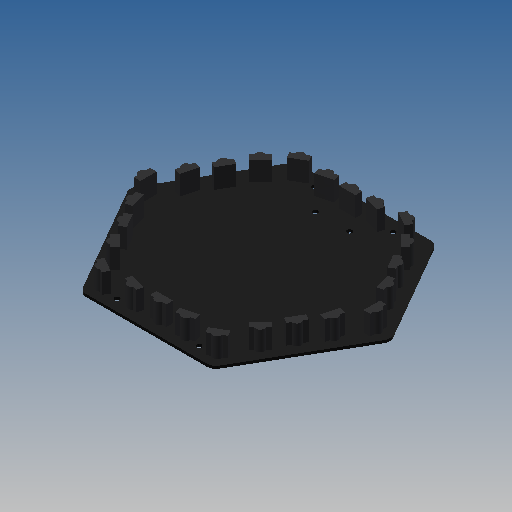
# Autodesk Inventor part: PCB
Saved by Autodesk Inventor 2017 (Build 210142000, 142)
## iProperties
Created: 2016-10-01
Part Number: PCB
Material: Generic
Document SubType Name: Modeling
Designer: James Yelland
Density: 1 g/cm^3
Appearance: Default
Mass: 32.3214 g
Surface Area: 333.79 cm^2
Volume: 32.3214 cm^3
Author: James Yelland
Autodesk Inventor part; units mm, degrees
ref_plane "YZ Plane" through (0, 0, 0) normal (1, 0, 0) x (0, 1, 0)
ref_plane "XZ Plane" through (0, 0, 0) normal (0, 1, 0) x (-1, 0, 0)
ref_plane "XY Plane" through (0, 0, 0) normal (0, 0, 1) x (1, 0, 0)
sketch "Sketch1" plane through (0, 0, 0) normal (0, 1, 0) x (-1, 0, 0)
  line L0 (-78.5566, 2.5) -> (-41.4434, 66.782)
  line L1 (-37.1132, 69.282) -> (37.1132, 69.282)
  line L2 (41.4434, 66.782) -> (78.5566, 2.5)
  line L3 (0, -64.282) -> (-40, -64.282)
  line L4 (0, -64.282) -> (40, -64.282)
  line L5 (78.5566, -2.5) -> (44.3301, -61.782)
  line L6 (-44.3301, -61.782) -> (-78.5566, -2.5)
  arc A0 (78.5566, -2.5) -> (78.5566, 2.5) centre (74.2265, 0) ccw
  arc A1 (40, -64.282) -> (44.3301, -61.782) centre (40, -59.282) ccw
  arc A2 (-44.3301, -61.782) -> (-40, -64.282) centre (-40, -59.282) ccw
  arc A3 (-78.5566, 2.5) -> (-78.5566, -2.5) centre (-74.2265, 0) ccw
  arc A4 (-37.1132, 69.282) -> (-41.4434, 66.782) centre (-37.1132, 64.282) ccw
  arc A5 (41.4434, 66.782) -> (37.1132, 69.282) centre (37.1132, 64.282) ccw
  point P0 (80, 0)
  point P1 (-80, 0)
  point P2 (-42.8868, -64.282)
  point P3 (42.8868, -64.282)
  dimension "d21" = 5
  constraints: 14 end point, 12 point on circle, 12 tangent, 9 point on line, 6 centre point, 5 equal radius
  measures "d21" radius of A0
extrude "Extrusion1" add sketch "Sketch1" along normal blind 1.6
sketch "Sketch4" plane through (0, 1.6, 0) normal (0, 1, 0) x (1, 0, 0)
  line L0 (5, 57.282) -> (5, 53.282)
  arc A0 (2.5807, 57.282) -> (-2.5807, 57.282) centre (0, 56.332) ccw
  line L1 (-5, 57.282) -> (-2.5807, 57.282)
  line L2 (5, 53.282) -> (-5, 53.282)
  line L3 (-5, 53.282) -> (-5, 57.282)
  line L4 (2.5807, 57.282) -> (5, 57.282)
  line L5 (40, 64.282) -> (-40, 64.282)
  arc A1 (-40, 64.282) -> (-44.3301, 61.782) centre (-40, 59.282) ccw
  line L6 (-44.3301, 61.782) -> (-78.5566, 2.5)
  arc A2 (-78.5566, 2.5) -> (-78.5566, -2.5) centre (-74.2265, 0) ccw
  line L7 (-78.5566, -2.5) -> (-41.4434, -66.782)
  arc A3 (-41.4434, -66.782) -> (-37.1132, -69.282) centre (-37.1132, -64.282) ccw
  line L8 (-37.1132, -69.282) -> (37.1132, -69.282)
  arc A4 (37.1132, -69.282) -> (41.4434, -66.782) centre (37.1132, -64.282) ccw
  line L9 (41.4434, -66.782) -> (78.5566, -2.5)
  arc A5 (78.5566, -2.5) -> (78.5566, 2.5) centre (74.2265, 0) ccw
  line L10 (78.5566, 2.5) -> (44.3301, 61.782)
  arc A6 (44.3301, 61.782) -> (40, 64.282) centre (40, 59.282) ccw
  line L11 (0, 56.332) -> (0, 64.282)
  line L12 (-19.2069, 52.3628) -> (-20.2422, 56.2265)
  line L13 (-20.2422, 56.2265) -> (-17.9053, 56.8526)
  arc A7 (-12.9198, 58.1885) -> (-17.9053, 56.8526) centre (-15.1667, 56.6029) ccw
  line L14 (-9.5477, 54.9509) -> (-19.2069, 52.3628)
  line L15 (-10.583, 58.8146) -> (-9.5477, 54.9509)
  line L16 (-12.9198, 58.1885) -> (-10.583, 58.8146)
  line L17 (-15.1667, 56.6029) -> (-17.2243, 64.282)
  line L18 (-35.9434, 52.2558) -> (-37.9434, 55.7199)
  line L19 (-37.9434, 55.7199) -> (-35.8482, 56.9295)
  arc A8 (-31.3783, 59.5102) -> (-35.8482, 56.9295) centre (-33.1382, 57.3971) ccw
  line L20 (-27.2831, 57.2558) -> (-35.9434, 52.2558)
  line L21 (-29.2831, 60.7199) -> (-27.2831, 57.2558)
  line L22 (-31.3783, 59.5102) -> (-29.2831, 60.7199)
  line L23 (-33.1382, 57.3971) -> (-37.1132, 64.282)
  line L24 (-46.4753, 39.4043) -> (-49.3038, 42.2327)
  line L25 (-49.3038, 42.2327) -> (-47.593, 43.9434)
  arc A9 (-43.9434, 47.593) -> (-47.593, 43.9434) centre (-45.0965, 45.0965) ccw
  line L26 (-39.4043, 46.4753) -> (-46.4753, 39.4043)
  line L27 (-42.2327, 49.3038) -> (-39.4043, 46.4753)
  line L28 (-43.9434, 47.593) -> (-42.2327, 49.3038)
  line L29 (-45.0965, 45.0965) -> (-50.718, 50.718)
  line L30 (-52.9737, 24.8109) -> (-56.4378, 26.8109)
  line L31 (-56.4378, 26.8109) -> (-55.2282, 28.9061)
  arc A10 (-52.6475, 33.376) -> (-55.2282, 28.9061) centre (-53.1151, 30.666) ccw
  line L32 (-47.9737, 33.4711) -> (-52.9737, 24.8109)
  line L33 (-51.4378, 35.4711) -> (-47.9737, 33.4711)
  line L34 (-52.6475, 33.376) -> (-51.4378, 35.4711)
  line L35 (-53.1151, 30.666) -> (-60, 34.641)
  line L36 (-59.9509, 10.8874) -> (-63.8146, 11.9227)
  line L37 (-63.8146, 11.9227) -> (-63.1885, 14.2596)
  arc A11 (-61.8526, 19.2451) -> (-63.1885, 14.2596) centre (-61.6029, 16.5065) ccw
  line L38 (-57.3628, 20.5467) -> (-59.9509, 10.8874)
  line L39 (-61.2265, 21.582) -> (-57.3628, 20.5467)
  line L40 (-61.8526, 19.2451) -> (-61.2265, 21.582)
  line L41 (-61.6029, 16.5065) -> (-69.282, 18.5641)
  line L42 (-68.2265, -5) -> (-72.2265, -5)
  line L43 (-72.2265, -5) -> (-72.2265, -2.5807)
  arc A12 (-72.2265, 2.5807) -> (-72.2265, -2.5807) centre (-71.2765, 0) ccw
  line L44 (-68.2265, 5) -> (-68.2265, -5)
  line L45 (-72.2265, 5) -> (-68.2265, 5)
  line L46 (-72.2265, 2.5807) -> (-72.2265, 5)
  line L47 (-71.2765, 0) -> (-79.2265, 0)
  line L48 (-57.3628, -20.5467) -> (-61.2265, -21.582)
  line L49 (-61.2265, -21.582) -> (-61.8526, -19.2451)
  arc A13 (-63.1885, -14.2596) -> (-61.8526, -19.2451) centre (-61.6029, -16.5065) ccw
  line L50 (-59.9509, -10.8874) -> (-57.3628, -20.5467)
  line L51 (-63.8146, -11.9227) -> (-59.9509, -10.8874)
  line L52 (-63.1885, -14.2596) -> (-63.8146, -11.9227)
  line L53 (-61.6029, -16.5065) -> (-69.282, -18.5641)
  line L54 (-47.9737, -33.4711) -> (-51.4378, -35.4711)
  line L55 (-51.4378, -35.4711) -> (-52.6475, -33.376)
  arc A14 (-55.2282, -28.9061) -> (-52.6475, -33.376) centre (-53.1151, -30.666) ccw
  line L56 (-52.9737, -24.8109) -> (-47.9737, -33.4711)
  line L57 (-56.4378, -26.8109) -> (-52.9737, -24.8109)
  line L58 (-55.2282, -28.9061) -> (-56.4378, -26.8109)
  line L59 (-53.1151, -30.666) -> (-60, -34.641)
  line L60 (-39.4043, -46.4753) -> (-42.2327, -49.3038)
  line L61 (-42.2327, -49.3038) -> (-43.9434, -47.593)
  arc A15 (-47.593, -43.9434) -> (-43.9434, -47.593) centre (-45.0965, -45.0965) ccw
  line L62 (-46.4753, -39.4043) -> (-39.4043, -46.4753)
  line L63 (-49.3038, -42.2327) -> (-46.4753, -39.4043)
  line L64 (-47.593, -43.9434) -> (-49.3038, -42.2327)
  line L65 (-45.0965, -45.0965) -> (-50.718, -50.718)
  line L66 (-29.7831, -61.5859) -> (-31.7831, -65.05)
  line L67 (-31.7831, -65.05) -> (-33.8783, -63.8403)
  arc A16 (-38.3482, -61.2596) -> (-33.8783, -63.8403) centre (-35.6382, -61.7273) ccw
  line L68 (-38.4434, -56.5859) -> (-29.7831, -61.5859)
  line L69 (-40.4434, -60.05) -> (-38.4434, -56.5859)
  line L70 (-38.3482, -61.2596) -> (-40.4434, -60.05)
  line L71 (-35.6382, -61.7273) -> (-39.6132, -68.6122)
  line L72 (-10.8874, -59.9509) -> (-11.9227, -63.8146)
  line L73 (-11.9227, -63.8146) -> (-14.2596, -63.1885)
  arc A17 (-19.2451, -61.8526) -> (-14.2596, -63.1885) centre (-16.5065, -61.6029) ccw
  line L74 (-20.5467, -57.3628) -> (-10.8874, -59.9509)
  line L75 (-21.582, -61.2265) -> (-20.5467, -57.3628)
  line L76 (-19.2451, -61.8526) -> (-21.582, -61.2265)
  line L77 (-16.5065, -61.6029) -> (-18.5641, -69.282)
  line L78 (5, -58.282) -> (5, -62.282)
  line L79 (5, -62.282) -> (2.5807, -62.282)
  arc A18 (-2.5807, -62.282) -> (2.5807, -62.282) centre (0, -61.332) ccw
  line L80 (-5, -58.282) -> (5, -58.282)
  line L81 (-5, -62.282) -> (-5, -58.282)
  line L82 (-2.5807, -62.282) -> (-5, -62.282)
  line L83 (0, -61.332) -> (0, -69.282)
  line L84 (20.5467, -57.3628) -> (21.582, -61.2265)
  line L85 (21.582, -61.2265) -> (19.2451, -61.8526)
  arc A19 (14.2596, -63.1885) -> (19.2451, -61.8526) centre (16.5065, -61.6029) ccw
  line L86 (10.8874, -59.9509) -> (20.5467, -57.3628)
  line L87 (11.9227, -63.8146) -> (10.8874, -59.9509)
  line L88 (14.2596, -63.1885) -> (11.9227, -63.8146)
  line L89 (16.5065, -61.6029) -> (18.5641, -69.282)
  line L90 (38.4434, -56.5859) -> (40.4434, -60.05)
  line L91 (40.4434, -60.05) -> (38.3482, -61.2596)
  arc A20 (33.8783, -63.8403) -> (38.3482, -61.2596) centre (35.6382, -61.7273) ccw
  line L92 (29.7831, -61.5859) -> (38.4434, -56.5859)
  line L93 (31.7831, -65.05) -> (29.7831, -61.5859)
  line L94 (33.8783, -63.8403) -> (31.7831, -65.05)
  line L95 (35.6382, -61.7273) -> (39.6132, -68.6122)
  line L96 (46.4753, -39.4043) -> (49.3038, -42.2327)
  line L97 (49.3038, -42.2327) -> (47.593, -43.9434)
  arc A21 (43.9434, -47.593) -> (47.593, -43.9434) centre (45.0965, -45.0965) ccw
  line L98 (39.4043, -46.4753) -> (46.4753, -39.4043)
  line L99 (42.2327, -49.3038) -> (39.4043, -46.4753)
  line L100 (43.9434, -47.593) -> (42.2327, -49.3038)
  line L101 (45.0965, -45.0965) -> (50.718, -50.718)
  line L102 (52.9737, -24.8109) -> (56.4378, -26.8109)
  line L103 (56.4378, -26.8109) -> (55.2282, -28.9061)
  arc A22 (52.6475, -33.376) -> (55.2282, -28.9061) centre (53.1151, -30.666) ccw
  line L104 (47.9737, -33.4711) -> (52.9737, -24.8109)
  line L105 (51.4378, -35.4711) -> (47.9737, -33.4711)
  line L106 (52.6475, -33.376) -> (51.4378, -35.4711)
  line L107 (53.1151, -30.666) -> (60, -34.641)
  line L108 (59.9509, -10.8874) -> (63.8146, -11.9227)
  line L109 (63.8146, -11.9227) -> (63.1885, -14.2596)
  arc A23 (61.8526, -19.2451) -> (63.1885, -14.2596) centre (61.6029, -16.5065) ccw
  line L110 (57.3628, -20.5467) -> (59.9509, -10.8874)
  line L111 (61.2265, -21.582) -> (57.3628, -20.5467)
  line L112 (61.8526, -19.2451) -> (61.2265, -21.582)
  line L113 (61.6029, -16.5065) -> (69.282, -18.5641)
  line L114 (68.2265, 5) -> (72.2265, 5)
  line L115 (72.2265, 5) -> (72.2265, 2.5807)
  arc A24 (72.2265, -2.5807) -> (72.2265, 2.5807) centre (71.2765, 0) ccw
  line L116 (68.2265, -5) -> (68.2265, 5)
  line L117 (72.2265, -5) -> (68.2265, -5)
  line L118 (72.2265, -2.5807) -> (72.2265, -5)
  line L119 (71.2765, 0) -> (79.2265, 0)
  line L120 (57.3628, 20.5467) -> (61.2265, 21.582)
  line L121 (61.2265, 21.582) -> (61.8526, 19.2451)
  arc A25 (63.1885, 14.2596) -> (61.8526, 19.2451) centre (61.6029, 16.5065) ccw
  line L122 (59.9509, 10.8874) -> (57.3628, 20.5467)
  line L123 (63.8146, 11.9227) -> (59.9509, 10.8874)
  line L124 (63.1885, 14.2596) -> (63.8146, 11.9227)
  line L125 (61.6029, 16.5065) -> (69.282, 18.5641)
  line L126 (47.9737, 33.4711) -> (51.4378, 35.4711)
  line L127 (51.4378, 35.4711) -> (52.6475, 33.376)
  arc A26 (55.2282, 28.9061) -> (52.6475, 33.376) centre (53.1151, 30.666) ccw
  line L128 (52.9737, 24.8109) -> (47.9737, 33.4711)
  line L129 (56.4378, 26.8109) -> (52.9737, 24.8109)
  line L130 (55.2282, 28.9061) -> (56.4378, 26.8109)
  line L131 (53.1151, 30.666) -> (60, 34.641)
  line L132 (39.4043, 46.4753) -> (42.2327, 49.3038)
  line L133 (42.2327, 49.3038) -> (43.9434, 47.593)
  arc A27 (47.593, 43.9434) -> (43.9434, 47.593) centre (45.0965, 45.0965) ccw
  line L134 (46.4753, 39.4043) -> (39.4043, 46.4753)
  line L135 (49.3038, 42.2327) -> (46.4753, 39.4043)
  line L136 (47.593, 43.9434) -> (49.3038, 42.2327)
  line L137 (45.0965, 45.0965) -> (50.718, 50.718)
  line L138 (27.2831, 57.2558) -> (29.2831, 60.7199)
  line L139 (29.2831, 60.7199) -> (31.3783, 59.5102)
  arc A28 (35.8482, 56.9295) -> (31.3783, 59.5102) centre (33.1382, 57.3971) ccw
  line L140 (35.9434, 52.2557) -> (27.2831, 57.2558)
  line L141 (37.9434, 55.7199) -> (35.9434, 52.2557)
  line L142 (35.8482, 56.9295) -> (37.9434, 55.7199)
  line L143 (33.1382, 57.3971) -> (37.1132, 64.282)
  line L144 (9.5477, 54.9509) -> (10.583, 58.8146)
  line L145 (10.583, 58.8146) -> (12.9198, 58.1885)
  arc A29 (17.9053, 56.8526) -> (12.9198, 58.1885) centre (15.1667, 56.6029) ccw
  line L146 (19.2069, 52.3628) -> (9.5477, 54.9509)
  line L147 (20.2422, 56.2265) -> (19.2069, 52.3628)
  line L148 (17.9053, 56.8526) -> (20.2422, 56.2265)
  line L149 (15.1667, 56.6029) -> (17.2243, 64.282)
  line L150 (40, 64.282) -> (-40, 64.282) projected
  line L151 (-78.5566, 2.5) -> (-44.3301, 61.782) projected
  arc A30 (-78.5566, 2.5) -> (-78.5566, -2.5) centre (-74.2265, 0) ccw projected
  line L152 (-41.4434, -66.782) -> (-78.5566, -2.5) projected
  arc A31 (-41.4434, -66.782) -> (-37.1132, -69.282) centre (-37.1132, -64.282) ccw projected
  line L153 (37.1132, -69.282) -> (-37.1132, -69.282) projected
  line L154 (78.5566, -2.5) -> (41.4434, -66.782) projected
  line L155 (78.5566, 2.5) -> (44.3301, 61.782) projected
  dimension "d24" = 360
  dimension "d49" = 360
  constraints: 300 end point, 60 point on circle, 36 centre point, 1 midpoint
extrude "Extrusion4" add sketch "Sketch4" along normal blind 12 contours L0 L2 L3 L1 A0 L4 | L12 L13 A7 L16 L15 L14 | L18 L19 A8 L22 L21 L20 | L24 L25 A9 L28 L27 L26 | L30 L31 A10 L34 L33 L32 | L36 L37 A11 L40 L39 L38 | L42 L43 A12 L46 L45 L44 | L48 L49 A13 L52 L51 L50 | L54 L55 A14 L58 L57 L56 | L60 L61 A15 L64 L63 L62 | L66 L67 A16 L70 L69 L68 | L72 L73 A17 L76 L75 L74 | L78 L79 A18 L82 L81 L80 | L84 L85 A19 L88 L87 L86 | L90 L91 A20 L94 L93 L92 | L96 L97 A21 L100 L99 L98 | L102 L103 A22 L106 L105 L104 | L108 L109 A23 L112 L111 L110 | L114 L115 A24 L118 L117 L116 | L120 L121 A25 L124 L123 L122 | L126 L127 A26 L130 L129 L128 | L132 L133 A27 L136 L135 L134 | L138 L139 A28 L142 L141 L140 | L144 L145 A29 L148 L147 L146
sketch "Sketch5" plane through (0, 1.6, 0) normal (0, 1, 0) x (1, 0, 0)
  line L0 (-37.1132, -69.282) -> (37.1132, -69.282) projected
  line L1 (0, -69.282) -> (25, -69.282)
  line L2 (25, -69.282) -> (25, -62.282)
  line L3 (0, -69.282) -> (-25, -69.282)
  line L4 (-25, -69.282) -> (-25, -62.282)
  circle A0 centre (25, -62.282) radius 1.6
  circle A1 centre (-25, -62.282) radius 1.6
  line L5 (40, 64.282) -> (-40, 64.282) projected
  line L6 (0, 64.282) -> (24, 64.282)
  line L7 (0, 64.282) -> (-24, 64.282)
  line L8 (-24, 64.282) -> (-24, 57.282)
  circle A2 centre (-24, 57.282) radius 1.6
  line L9 (24, 64.282) -> (24, 57.282)
  circle A3 centre (24, 57.282) radius 1.6
  line L10 (0, 64.282) -> (0, 44.282)
  circle A4 centre (-10.414, 44.282) radius 1.6
  circle A5 centre (10.414, 44.282) radius 1.6
  line L11 (-10.414, 44.282) -> (10.414, 44.282)
  point P0 (0, 0)
  dimension "d56" = 25
  dimension "d57" = 7
  dimension "d58" = 90
  dimension "d59" = 25
  dimension "d60" = 7
  dimension "d61" = 90
  dimension "d62" = 3.2
  dimension "d63" = 3.2
  dimension "d64" = 24
  dimension "d65" = 24
  dimension "d66" = 7
  dimension "d67" = 3.2
  dimension "d68" = 7
  dimension "d69" = 3.2
  dimension "d81" = 20
  dimension "d82" = 3.2
  dimension "d83" = 3.2
  dimension "d84" = 0
  constraints: 20 end point, 6 centre point, 4 coincident, 4 point on line, 3 vertical, 2 midpoint, 2 perpendicular, 1 horizontal
  measures "d56" distance of L1.start L1.end
  measures "d57" distance of L1.end L2.end
  measures "d58" angle of L2 L1
  measures "d59" distance of L1.start L3.end
  measures "d60" distance of L3.end L4.end
  measures "d61" angle of L3 L4
  measures "d62" diameter of A0
  measures "d63" diameter of A1
  measures "d64" distance of L6.start L6.end
  measures "d65" distance of L6.start L7.end
  measures "d66" distance of L7.end L8.end
  measures "d67" diameter of A2
  measures "d68" distance of L6.end L9.end
  measures "d69" diameter of A3
  measures "d81" distance of L6.start L10.end
  measures "d82" diameter of A5
  measures "d83" diameter of A4
  measures "d84" distance from line of L10.end L11
extrude "Extrusion5" cut sketch "Sketch5" against normal through all
sketch "Sketch9" plane through (0, 1.6, 0) normal (0, 1, 0) x (1, 0, 0)
  circle A0 centre (-24, 57.282) radius 1.6
  circle A1 centre (25, -62.282) radius 1.6
  circle A2 centre (-25, -62.282) radius 1.6
  circle A3 centre (24, 57.282) radius 1.6
  line L0 (29.2831, 60.7199) -> (31.3783, 59.5102)
  arc A4 (35.8482, 56.9295) -> (31.3783, 59.5102) centre (33.1382, 57.3971) ccw
  line L1 (35.8482, 56.9295) -> (37.9434, 55.7199)
  line L2 (37.9434, 55.7199) -> (35.9434, 52.2557)
  line L3 (35.9434, 52.2557) -> (27.2831, 57.2558)
  line L4 (27.2831, 57.2558) -> (29.2831, 60.7199)
  line L5 (51.4378, 35.4711) -> (52.6475, 33.376)
  arc A5 (55.2282, 28.9061) -> (52.6475, 33.376) centre (53.1151, 30.666) ccw
  line L6 (55.2282, 28.9061) -> (56.4378, 26.8109)
  line L7 (56.4378, 26.8109) -> (52.9737, 24.8109)
  line L8 (52.9737, 24.8109) -> (47.9737, 33.4711)
  line L9 (47.9737, 33.4711) -> (51.4378, 35.4711)
  line L10 (72.2265, 5) -> (72.2265, 2.5807)
  arc A6 (72.2265, -2.5807) -> (72.2265, 2.5807) centre (71.2765, 0) ccw
  line L11 (72.2265, -2.5807) -> (72.2265, -5)
  line L12 (72.2265, -5) -> (68.2265, -5)
  line L13 (68.2265, -5) -> (68.2265, 5)
  line L14 (68.2265, 5) -> (72.2265, 5)
  line L15 (56.4378, -26.8109) -> (55.2282, -28.9061)
  arc A7 (52.6475, -33.376) -> (55.2282, -28.9061) centre (53.1151, -30.666) ccw
  line L16 (52.6475, -33.376) -> (51.4378, -35.4711)
  line L17 (51.4378, -35.4711) -> (47.9737, -33.4711)
  line L18 (47.9737, -33.4711) -> (52.9737, -24.8109)
  line L19 (52.9737, -24.8109) -> (56.4378, -26.8109)
  line L20 (40.4434, -60.05) -> (38.3482, -61.2596)
  arc A8 (33.8783, -63.8403) -> (38.3482, -61.2596) centre (35.6382, -61.7273) ccw
  line L21 (33.8783, -63.8403) -> (31.7831, -65.05)
  line L22 (31.7831, -65.05) -> (29.7831, -61.5859)
  line L23 (29.7831, -61.5859) -> (38.4434, -56.5859)
  line L24 (38.4434, -56.5859) -> (40.4434, -60.05)
  line L25 (5, -62.282) -> (2.5807, -62.282)
  arc A9 (-2.5807, -62.282) -> (2.5807, -62.282) centre (0, -61.332) ccw
  line L26 (-2.5807, -62.282) -> (-5, -62.282)
  line L27 (-5, -62.282) -> (-5, -58.282)
  line L28 (-5, -58.282) -> (5, -58.282)
  line L29 (5, -58.282) -> (5, -62.282)
  line L30 (-31.7831, -65.05) -> (-33.8783, -63.8403)
  arc A10 (-38.3482, -61.2596) -> (-33.8783, -63.8403) centre (-35.6382, -61.7273) ccw
  line L31 (-38.3482, -61.2596) -> (-40.4434, -60.05)
  line L32 (-40.4434, -60.05) -> (-38.4434, -56.5859)
  line L33 (-38.4434, -56.5859) -> (-29.7831, -61.5859)
  line L34 (-29.7831, -61.5859) -> (-31.7831, -65.05)
  line L35 (-51.4378, -35.4711) -> (-52.6475, -33.376)
  arc A11 (-55.2282, -28.9061) -> (-52.6475, -33.376) centre (-53.1151, -30.666) ccw
  line L36 (-55.2282, -28.9061) -> (-56.4378, -26.8109)
  line L37 (-56.4378, -26.8109) -> (-52.9737, -24.8109)
  line L38 (-52.9737, -24.8109) -> (-47.9737, -33.4711)
  line L39 (-47.9737, -33.4711) -> (-51.4378, -35.4711)
  line L40 (-72.2265, -5) -> (-72.2265, -2.5807)
  arc A12 (-72.2265, 2.5807) -> (-72.2265, -2.5807) centre (-71.2765, 0) ccw
  line L41 (-72.2265, 2.5807) -> (-72.2265, 5)
  line L42 (-72.2265, 5) -> (-68.2265, 5)
  line L43 (-68.2265, 5) -> (-68.2265, -5)
  line L44 (-68.2265, -5) -> (-72.2265, -5)
  line L45 (-56.4378, 26.8109) -> (-55.2282, 28.9061)
  arc A13 (-52.6475, 33.376) -> (-55.2282, 28.9061) centre (-53.1151, 30.666) ccw
  line L46 (-52.6475, 33.376) -> (-51.4378, 35.4711)
  line L47 (-51.4378, 35.4711) -> (-47.9737, 33.4711)
  line L48 (-47.9737, 33.4711) -> (-52.9737, 24.8109)
  line L49 (-52.9737, 24.8109) -> (-56.4378, 26.8109)
  line L50 (-37.9434, 55.7199) -> (-35.8482, 56.9295)
  arc A14 (-31.3783, 59.5102) -> (-35.8482, 56.9295) centre (-33.1382, 57.3971) ccw
  line L51 (-31.3783, 59.5102) -> (-29.2831, 60.7199)
  line L52 (-29.2831, 60.7199) -> (-27.2831, 57.2558)
  line L53 (-27.2831, 57.2558) -> (-35.9434, 52.2558)
  line L54 (-35.9434, 52.2558) -> (-37.9434, 55.7199)
  line L55 (-5, 57.282) -> (-2.5807, 57.282)
  arc A15 (2.5807, 57.282) -> (-2.5807, 57.282) centre (0, 56.332) ccw
  line L56 (2.5807, 57.282) -> (5, 57.282)
  line L57 (5, 57.282) -> (5, 53.282)
  line L58 (5, 53.282) -> (-5, 53.282)
  line L59 (-5, 53.282) -> (-5, 57.282)
  line L60 (-20.2422, 56.2265) -> (-17.9053, 56.8526)
  arc A16 (-12.9198, 58.1885) -> (-17.9053, 56.8526) centre (-15.1667, 56.6029) ccw
  line L61 (-12.9198, 58.1885) -> (-10.583, 58.8146)
  line L62 (-10.583, 58.8146) -> (-9.5477, 54.9509)
  line L63 (-9.5477, 54.9509) -> (-19.2069, 52.3628)
  line L64 (-19.2069, 52.3628) -> (-20.2422, 56.2265)
  line L65 (-49.3038, 42.2327) -> (-47.593, 43.9434)
  arc A17 (-43.9434, 47.593) -> (-47.593, 43.9434) centre (-45.0965, 45.0965) ccw
  line L66 (-43.9434, 47.593) -> (-42.2327, 49.3038)
  line L67 (-42.2327, 49.3038) -> (-39.4043, 46.4753)
  line L68 (-39.4043, 46.4753) -> (-46.4753, 39.4043)
  line L69 (-46.4753, 39.4043) -> (-49.3038, 42.2327)
  line L70 (-63.8146, 11.9227) -> (-63.1885, 14.2596)
  arc A18 (-61.8526, 19.2451) -> (-63.1885, 14.2596) centre (-61.6029, 16.5065) ccw
  line L71 (-61.8526, 19.2451) -> (-61.2265, 21.582)
  line L72 (-61.2265, 21.582) -> (-57.3628, 20.5467)
  line L73 (-57.3628, 20.5467) -> (-59.9509, 10.8874)
  line L74 (-59.9509, 10.8874) -> (-63.8146, 11.9227)
  line L75 (-61.2265, -21.582) -> (-61.8526, -19.2451)
  arc A19 (-63.1885, -14.2596) -> (-61.8526, -19.2451) centre (-61.6029, -16.5065) ccw
  line L76 (-63.1885, -14.2596) -> (-63.8146, -11.9227)
  line L77 (-63.8146, -11.9227) -> (-59.9509, -10.8874)
  line L78 (-59.9509, -10.8874) -> (-57.3628, -20.5467)
  line L79 (-57.3628, -20.5467) -> (-61.2265, -21.582)
  line L80 (-42.2327, -49.3038) -> (-43.9434, -47.593)
  arc A20 (-47.593, -43.9434) -> (-43.9434, -47.593) centre (-45.0965, -45.0965) ccw
  line L81 (-47.593, -43.9434) -> (-49.3038, -42.2327)
  line L82 (-49.3038, -42.2327) -> (-46.4753, -39.4043)
  line L83 (-46.4753, -39.4043) -> (-39.4043, -46.4753)
  line L84 (-39.4043, -46.4753) -> (-42.2327, -49.3038)
  line L85 (-11.9227, -63.8146) -> (-14.2596, -63.1885)
  arc A21 (-19.2451, -61.8526) -> (-14.2596, -63.1885) centre (-16.5065, -61.6029) ccw
  line L86 (-19.2451, -61.8526) -> (-21.582, -61.2265)
  line L87 (-21.582, -61.2265) -> (-20.5467, -57.3628)
  line L88 (-20.5467, -57.3628) -> (-10.8874, -59.9509)
  line L89 (-10.8874, -59.9509) -> (-11.9227, -63.8146)
  line L90 (21.582, -61.2265) -> (19.2451, -61.8526)
  arc A22 (14.2596, -63.1885) -> (19.2451, -61.8526) centre (16.5065, -61.6029) ccw
  line L91 (14.2596, -63.1885) -> (11.9227, -63.8146)
  line L92 (11.9227, -63.8146) -> (10.8874, -59.9509)
  line L93 (10.8874, -59.9509) -> (20.5467, -57.3628)
  line L94 (20.5467, -57.3628) -> (21.582, -61.2265)
  line L95 (49.3038, -42.2327) -> (47.593, -43.9434)
  arc A23 (43.9434, -47.593) -> (47.593, -43.9434) centre (45.0965, -45.0965) ccw
  line L96 (43.9434, -47.593) -> (42.2327, -49.3038)
  line L97 (42.2327, -49.3038) -> (39.4043, -46.4753)
  line L98 (39.4043, -46.4753) -> (46.4753, -39.4043)
  line L99 (46.4753, -39.4043) -> (49.3038, -42.2327)
  line L100 (63.8146, -11.9227) -> (63.1885, -14.2596)
  arc A24 (61.8526, -19.2451) -> (63.1885, -14.2596) centre (61.6029, -16.5065) ccw
  line L101 (61.8526, -19.2451) -> (61.2265, -21.582)
  line L102 (61.2265, -21.582) -> (57.3628, -20.5467)
  line L103 (57.3628, -20.5467) -> (59.9509, -10.8874)
  line L104 (59.9509, -10.8874) -> (63.8146, -11.9227)
  line L105 (61.2265, 21.582) -> (61.8526, 19.2451)
  arc A25 (63.1885, 14.2596) -> (61.8526, 19.2451) centre (61.6029, 16.5065) ccw
  line L106 (63.1885, 14.2596) -> (63.8146, 11.9227)
  line L107 (63.8146, 11.9227) -> (59.9509, 10.8874)
  line L108 (59.9509, 10.8874) -> (57.3628, 20.5467)
  line L109 (57.3628, 20.5467) -> (61.2265, 21.582)
  line L110 (42.2327, 49.3038) -> (43.9434, 47.593)
  arc A26 (47.593, 43.9434) -> (43.9434, 47.593) centre (45.0965, 45.0965) ccw
  line L111 (47.593, 43.9434) -> (49.3038, 42.2327)
  line L112 (49.3038, 42.2327) -> (46.4753, 39.4043)
  line L113 (46.4753, 39.4043) -> (39.4043, 46.4753)
  line L114 (39.4043, 46.4753) -> (42.2327, 49.3038)
  line L115 (10.583, 58.8146) -> (12.9198, 58.1885)
  arc A27 (17.9053, 56.8526) -> (12.9198, 58.1885) centre (15.1667, 56.6029) ccw
  line L116 (17.9053, 56.8526) -> (20.2422, 56.2265)
  line L117 (20.2422, 56.2265) -> (19.2069, 52.3628)
  line L118 (19.2069, 52.3628) -> (9.5477, 54.9509)
  line L119 (9.5477, 54.9509) -> (10.583, 58.8146)
  line L120 (40, 64.282) -> (-40, 64.282)
  arc A28 (-40, 64.282) -> (-44.3301, 61.782) centre (-40, 59.282) ccw
  line L121 (-44.3301, 61.782) -> (-78.5566, 2.5)
  arc A29 (-78.5566, 2.5) -> (-78.5566, -2.5) centre (-74.2265, 0) ccw
  line L122 (-78.5566, -2.5) -> (-41.4434, -66.782)
  arc A30 (-41.4434, -66.782) -> (-37.1132, -69.282) centre (-37.1132, -64.282) ccw
  line L123 (-37.1132, -69.282) -> (37.1132, -69.282)
  arc A31 (37.1132, -69.282) -> (41.4434, -66.782) centre (37.1132, -64.282) ccw
  line L124 (41.4434, -66.782) -> (78.5566, -2.5)
  arc A32 (78.5566, -2.5) -> (78.5566, 2.5) centre (74.2265, 0) ccw
  line L125 (78.5566, 2.5) -> (44.3301, 61.782)
  arc A33 (44.3301, 61.782) -> (40, 64.282) centre (40, 59.282) ccw
  line L126 (-47.0096, 27.141) -> (-35.6699, 46.782)
  line L127 (0, 49.282) -> (31.3397, 49.282)
  line L128 (47.0096, 27.141) -> (61.2361, 2.5)
  line L129 (47.0096, -27.141) -> (32.7831, -51.782)
  line L130 (-47.0096, -27.141) -> (-32.7831, -51.782)
  line L131 (-47.0096, -27.141) -> (-61.2361, -2.5)
  line L132 (-28.453, -54.282) -> (0, -54.282)
  line L133 (0, -54.282) -> (28.453, -54.282)
  line L134 (-61.2361, 2.5) -> (-47.0096, 27.141)
  line L135 (-31.3397, 49.282) -> (0, 49.282)
  line L136 (35.6699, 46.782) -> (47.0096, 27.141)
  line L137 (47.0096, -27.141) -> (61.2361, -2.5)
  arc A34 (-31.3397, 49.282) -> (-35.6699, 46.782) centre (-31.3397, 44.282) ccw
  arc A35 (35.6699, 46.782) -> (31.3397, 49.282) centre (31.3397, 44.282) ccw
  arc A36 (61.2361, -2.5) -> (61.2361, 2.5) centre (56.906, 0) ccw
  arc A37 (28.453, -54.282) -> (32.7831, -51.782) centre (28.453, -49.282) ccw
  arc A38 (-32.7831, -51.782) -> (-28.453, -54.282) centre (-28.453, -49.282) ccw
  arc A39 (-61.2361, 2.5) -> (-61.2361, -2.5) centre (-56.906, 0) ccw
  circle A40 centre (10.414, 44.282) radius 1.6 projected
  circle A41 centre (10.414, 44.282) radius 1.6 projected
  circle A42 centre (-10.414, 44.282) radius 1.6 projected
  point P0 (0, 0)
  constraints: 276 end point, 74 centre point, 72 point on circle
body "Solid1"
